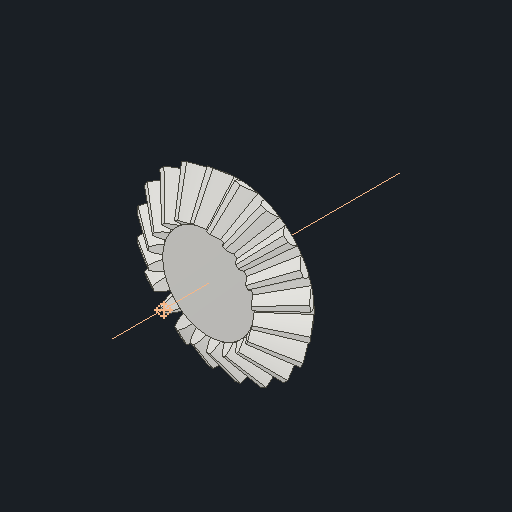
# Autodesk Inventor part: 베벨 기어1
Saved by Autodesk Inventor 2026.1 (Build 301233020, 233B)
## iProperties
Created: 2025-11-23
Part Number: 베벨 기어1
Material: Steel, Mild
Document SubType Name: Modeling
Designer: jaewook
Categories: <?xml version="1.0" encoding="UTF-16"?> <MemberInstance><Categories><FamilyTemplate><FamilyTemplateParameter ValueType="xs:double" Id="1" ObjectReferenceKey="da_z" ObjectType="kUserParameterObject"/><FamilyTemplateParameter ValueType="xs:double" Id="2" ObjectReferenceKey="da_b" ObjectType="kUserParameterObject"/><FamilyTemplateParameter ValueType="xs:double" Id="3" ObjectReferenceKey="da_beta" ObjectType="kUserParameterObject"/><FamilyTemplateParameter ValueType="xs:double" Id="4" ObjectReferenceKey="da_dae" ObjectType="kUserParameterObject"/><FamilyTemplateParameter ValueType="xs:double" Id="5" ObjectReferenceKey="da_ve" ObjectType="kUserParameterObject"/><FamilyTemplateParameter ValueType="xs:double" Id="6" ObjectReferenceKey="da_omega" ObjectType="kUserParameterObject"/><FamilyTemplateParameter ValueType="xs:string" Id="7" ObjectReferenceKey="EAIAABAAAAAAHwAAAAAAAIAAAAAAAAAA" ObjectType="83914240" SubObjectId="SurfaceGeometry"/></FamilyTemplate><ParamToTemplateMap><ParamToTemplate CategoryParameter="//CategoryParameter[@InternalName='046C89C9-8512-4d59-83FE-43B91F4F132A']" TemplateParameter="1"/><ParamToTemplate CategoryParameter="//CategoryParameter[@InternalName='2552DF32-E462-4b46-AEBF-C6C7768E72AC']" TemplateParameter="2"/><ParamToTemplate CategoryParameter="//CategoryParameter[@InternalName='C9EE641D-15FC-4fae-A226-E94C4372FDD7']" TemplateParameter="3"/><ParamToTemplate><ParamToTemplate CategoryParameter="//CategoryParameter[@InternalName='00B6519A-459B-49c7-AD84-2E56D39A5744']" ConstantValue="0.000000"/></ParamToTemplate><ParamToTemplate><ParamToTemplate CategoryParameter="//CategoryParameter[@InternalName='04B31F0E-C7A6-4894-AA32-9629BEFACF47']" ConstantValue="1.000000"/></ParamToTemplate><ParamToTemplate><ParamToTemplate CategoryParameter="//CategoryParameter[@InternalName='43CBEC2E-7847-49e7-A936-2F7889FCB2D9']" ConstantValue="0.200000"/></ParamToTemplate><ParamToTemplate><ParamToTemplate CategoryParameter="//CategoryParameter[@InternalName='B1EFC894-105D-4ebd-86BF-FA20ED196853']" ConstantValue="0.300000"/></ParamToTemplate><ParamToTemplate><ParamToTemplate CategoryParameter="//CategoryParameter[@InternalName='51175063-3D10-4879-93E8-6246FE8B403D']" ConstantValue="2060000000.000000"/></ParamToTemplate><ParamToTemplate><ParamToTemplate CategoryParameter="//CategoryParameter[@InternalName='A3A52E27-4454-46a9-B0BD-C932399B70AF']" ConstantValue="0.300000"/></ParamToTemplate><ParamToTemplate CategoryParameter="//CategoryParameter[@InternalName='2A200944-5A8C-41ca-B96E-8520D2E510F1']" TemplateParameter="4"/><ParamToTemplate><ParamToTemplate CategoryParameter="//CategoryParameter[@InternalName='1A637F62-92C8-44bc-B81F-10802510B579']" ConstantValue="1.594223"/></ParamToTemplate><ParamToTemplate CategoryParameter="//CategoryParameter[@InternalName='B52DD4BE-6863-48fb-BF58-89EF6F9EC65C']" TemplateParameter="5"/><ParamToTemplate><ParamToTemplate CategoryParameter="//CategoryParameter[@InternalName='3956BFF2-84D2-457d-93C2-9B0613DEBA67']" ConstantValue="0.541611"/></ParamToTemplate><ParamToTemplate CategoryParameter="//CategoryParameter[@InternalName='739CFA02-461B-4bf8-8049-181FCAD8B28F']" TemplateParameter="6"/><ParamToTemplate><ParamToTemplate CategoryParameter="//CategoryParameter[@InternalName='A27E999F-E2CE-4481-8A2A-EBF499C4C3C5']" ConstantValue="0.000000"/></ParamToTemplate><ParamToTemplate><ParamToTemplate CategoryParameter="//CategoryParameter[@InternalName='9E1B4470-B2D3-4ff1-B813-535BB4CDF51A']" ConstantValue="3520000.000000"/></ParamToTemplate><ParamToTemplate><ParamToTemplate CategoryParameter="//CategoryParameter[@InternalName='F8452263-BFF6-458c-9FB1-07C4B99E95CD']" ConstantValue="11400000.000000"/></ParamToTemplate><ParamToTemplate><ParamToTemplate CategoryParameter="//CategoryParameter[@InternalName='3E3BB259-FD49-497f-8171-6EBC954A3479']" ConstantValue="2.000000"/></ParamToTemplate><ParamToTemplate CategoryParameter="//CategoryParameter[@InternalName='27C3BAF2-7550-4e4b-AE2C-0DB134B7D9B7']" TemplateParameter="7"/></ParamToTemplateMap><Category DisplayName="Gear" InternalName="DC85795E-93AB-48d5-8EEE-5A27447B64BD" Mnemonic="Gear"><CategoryParameter DisplayName="z" InternalName="046C89C9-8512-4d59-83FE-43B91F4F132A" Mnemonic="z"/><CategoryParameter DisplayName="b" InternalName="2552DF32-E462-4b46-AEBF-C6C7768E72AC" Mnemonic="b"/><CategoryParameter DisplayName="||b|" InternalName="C9EE641D-15FC-4fae-A226-E94C4372FDD7" Mnemonic="beta"/><CategoryParameter DisplayName="x" InternalName="00B6519A-459B-49c7-AD84-2E56D39A5744" Mnemonic="x"/><CategoryParameter DisplayName="a*" InternalName="04B31F0E-C7A6-4894-AA32-9629BEFACF47" Mnemonic="a"/><CategoryParameter DisplayName="c*" InternalName="43CBEC2E-7847-49e7-A936-2F7889FCB2D9" Mnemonic="c"/><CategoryParameter DisplayName="r|.f|*" InternalName="B1EFC894-105D-4ebd-86BF-FA20ED196853" Mnemonic="rf"/><CategoryParameter DisplayName="E" InternalName="51175063-3D10-4879-93E8-6246FE8B403D" Mnemonic="E"/><CategoryParameter DisplayName="||m|" InternalName="A3A52E27-4454-46a9-B0BD-C932399B70AF" Mnemonic="mi"/><Category DisplayName="BevelGear" InternalName="0C98F69A-0C2B-4791-B2FE-7691BB227E77" Mnemonic="BevelGear"><CategoryParameter DisplayName="d|.ae|" InternalName="2A200944-5A8C-41ca-B96E-8520D2E510F1" Mnemonic="dae"/><CategoryParameter DisplayName="d|.ai|" InternalName="1A637F62-92C8-44bc-B81F-10802510B579" Mnemonic="dai"/><CategoryParameter DisplayName="A|.e|" InternalName="B52DD4BE-6863-48fb-BF58-89EF6F9EC65C" Mnemonic="ve"/><CategoryParameter DisplayName="A|.i|" InternalName="3956BFF2-84D2-457d-93C2-9B0613DEBA67" Mnemonic="vi"/><CategoryParameter DisplayName="||S|" InternalName="739CFA02-461B-4bf8-8049-181FCAD8B28F" Mnemonic="omega"/><CategoryParameter DisplayName="x|.t|" InternalName="A27E999F-E2CE-4481-8A2A-EBF499C4C3C5" Mnemonic="xt"/><CategoryParameter DisplayName="||s||.Flim|" InternalName="9E1B4470-B2D3-4ff1-B813-535BB4CDF51A" Mnemonic="sFlim"/><CategoryParameter DisplayName="||s||.Hlim|" InternalName="F8452263-BFF6-458c-9FB1-07C4B99E95CD" Mnemonic="sHlim"/><CategoryParameter DisplayName="유형" InternalName="3E3BB259-FD49-497f-8171-6EBC954A3479" Mnemonic="type"/><CategoryParameter DisplayName="PitchDiameter" InternalName="27C3BAF2-7550-4e4b-AE2C-0DB134B7D9B7" Mnemonic="IDS_PITCHDIAM"/></Category></Category></Categories></MemberInstance>
Mass: 60.9118 g
Surface Area: 34.3074 cm^2
Volume: 7.7496 cm^3
Density: 7.86 g/cm^3
Appearance: Steel
CustomPartVersion: 1
Author: jaewook
Autodesk Inventor part; units mm, degrees
ref_plane "메쉬 평면2" through (0, 0, 0) normal (0.9876883, 0.1564345, 0) x (0, 0, 1)
sketch "톱니 본체 스케치" plane through (0, 0, 0) normal (1, 0, 0) x (0, 1, 0)
  line L0 (0, 0) -> (11.562957, -11.171303) construction
  line L1 (11.562957, -11.171303) -> (13.280869, -9.023914)
  line L2 (13.280869, -9.023914) -> (0, 0) construction
  line L3 (12.5, -10) -> (0, 0) construction
  line L4 (6.940031, -6.704962) -> (7.971113, -5.41611)
  line L5 (11.562957, -11.171303) -> (6.940031, -6.704962)
  line L6 (13.280869, -9.023914) -> (7.971113, -5.41611)
  line L7 (0, -39.386751) -> (0, 6.564458)
  line L8 (0, -10) -> (13.280869, -10) construction
  dimension "d0" = 25
  dimension "d1" = 23.12591
  dimension "d2" = 26.56174
  dimension "d3" = 6.4
  dimension "d4" = 9.02391
  constraints: 16 end point, 4 point on line, 3 perpendicular, 2 collinear, 1 horizontal alignment, 1 vertical alignment
  measures "d0" diameter of L3.start L7
  measures "d1" diameter of L0.end L7
  measures "d2" diameter of L1.end L7
  measures "d3" distance between parallel lines of L1 L4
  measures "d4" vertical distance of L1.end L0.start
revolve "톱니 본체" add sketch "톱니 본체 스케치" angle 360 about axis through (0, 0, 0) along (0, 0, 1)
ref_plane "톱니 평면" through (0, 12.5, -10) normal (0, -0.7808688, 0.624695) x (1, 0, 0)
sketch "시작 스케치" plane through (0, 12.5, -10) normal (0, -0.7808688, 0.624695) x (1, 0, 0)
  line L0 (0, -23.505131) -> (0, 10.644758)
  arc A0 (-0.488954, -1.83) -> (-2.245942, 1.960501) centre (-7.685775, -2.863445) ccw
  arc A1 (2.245942, 1.960501) -> (0.488954, -1.83) centre (7.685775, -2.863445) ccw
  line L1 (-0.488954, -1.83) -> (0.488954, -1.83)
  arc A2 (2.245942, 1.960501) -> (-2.245942, 1.960501) centre (0, -20.009763) ccw
  dimension "d7" = 7.27064
  dimension "d8" = 7.68577
  dimension "d9" = 17.14632
  dimension "d57" = 22.08476
  dimension "d58" = 18.17976
  constraints: 6 point on circle, 3 centre point, 3 symmetric about line, 2 end point, 1 coincident, 1 perpendicular, 1 other
  measures "d7" radius of A0
  measures "d8" horizontal distance of point (0, -20.01) A0.centre
  measures "d9" vertical distance of point (0, -20.01) A0.centre
  measures "d57" radius of A2
  measures "d58" distance from line of A2.centre L1
ref_plane "끝 평면" through (0, 7.39507, -5.916056) normal (0, -0.7808688, 0.624695) x (1, 0, 0)
sketch "끝 스케치" plane through (0, 7.39507, -5.916056) normal (0, -0.7808688, 0.624695) x (1, 0, 0)
  line L0 (0, -15.35404) -> (0, 6.953444)
  arc A0 (-0.289268, -1.082638) -> (-1.328712, 1.159843) centre (-4.546948, -1.69403) ccw
  arc A1 (1.328712, 1.159843) -> (0.289268, -1.082638) centre (4.546948, -1.69403) ccw
  line L1 (-0.289268, -1.082638) -> (0.289268, -1.082638)
  arc A2 (1.328712, 1.159843) -> (-1.328712, 1.159843) centre (0, -11.837888) ccw
  dimension "d12" = 4.30135
  dimension "d15" = 4.54695
  dimension "d16" = 10.14386
  dimension "d59" = 13.06547
  dimension "d60" = 10.75525
  constraints: 6 point on circle, 3 centre point, 3 symmetric about line, 2 end point, 1 coincident, 1 other
  measures "d12" radius of A0
  measures "d15" horizontal distance of A0.centre point (0, -11.838)
  measures "d16" vertical distance of A0.centre point (0, -11.838)
  measures "d59" radius of A2
  measures "d60" distance from line of A2.centre L1
loft "Loft" cut profiles "시작 스케치", "끝 스케치"
pattern_circular "Circular Pattern" count 20 over 360 about axis through (0, 0, 0) along (0, 0, 1) of "Loft"
sketch3d "3D 스케치 오른쪽"
ref_plane "끝 평면 오른쪽" through (-1.742858, 7.186759, -5.916056) normal (0.1840339, -0.7588726, 0.624695) x (0.9718311, 0.2356783, 0)
sketch "끝 스케치 오른쪽" plane through (-1.742858, 7.186759, -5.916056) normal (0.1840339, -0.7588726, 0.624695) x (0.9718311, 0.2356783, 0)
  arc A0 (-0.289268, -1.082638) -> (-1.328712, 1.159843) centre (-4.546948, -1.69403) ccw
  line L0 (0, -17.993564) -> (0, 9.592957)
  arc A1 (1.328712, 1.159843) -> (0.289268, -1.082638) centre (4.546948, -1.69403) ccw
  line L1 (-0.289268, -1.082638) -> (0.289268, -1.082638)
  arc A2 (1.328712, 1.159843) -> (-1.328712, 1.159843) centre (0, -11.837888) ccw
  dimension "d70" = 4.54695
  dimension "d71" = 10.14386
  dimension "d72" = 4.30135
  dimension "d73" = 10.75525
  dimension "d74" = 13.06547
  constraints: 6 point on circle, 3 centre point, 3 symmetric about line, 2 end point, 1 coincident, 1 perpendicular, 1 other
  measures "d70" horizontal distance of A2.centre A0.centre
  measures "d71" vertical distance of point (0, -11.838) A0.centre
  measures "d72" radius of A0
  measures "d73" distance from line of point (0, -11.838) L1
  measures "d74" radius of A2
feature "로프트 오른쪽" [suppressed]
pattern_circular "원형 패턴 오른쪽" [suppressed]
sketch3d "3D 스케치 왼쪽"
ref_plane "끝 평면 왼쪽" through (1.76116, 7.186759, -5.923915) normal (-0.1858037, -0.7582085, 0.6249775) x (0.9712618, -0.2380138, 0)
sketch "끝 스케치 왼쪽" plane through (1.76116, 7.186759, -5.923915) normal (-0.1858037, -0.7582085, 0.6249775) x (0.9712618, -0.2380138, 0)
  line L0 (0, -31.02314) -> (0, 14.000417)
  arc A0 (-0.289268, -1.079211) -> (-1.328712, 1.16327) centre (-4.546948, -1.690603) ccw
  arc A1 (1.328712, 1.16327) -> (0.289268, -1.079211) centre (4.546948, -1.690603) ccw
  line L1 (-0.289268, -1.079211) -> (0.289268, -1.079211)
  ellipse E0 centre (0, -4.228047) end of major axis (7.971113, -4.228047) minor radius 4.981766
  arc A2 (1.328712, 1.16327) -> (-1.328712, 1.16327) centre (0, -11.834461) ccw
  dimension "d56" = 4.98177
  dimension "d30" = 4.30135
  dimension "d31" = 4.54695
  dimension "d32" = 10.14386
  dimension "d61" = 13.06547
  dimension "d62" = 10.75525
  constraints: 6 point on circle, 3 centre point, 3 symmetric about line, 2 end point, 1 coincident, 2 other
  measures "d30" radius of A0
  measures "d31" horizontal distance of point (0, -11.834) A0.centre
  measures "d32" vertical distance of A0.centre point (0, -11.834)
  measures "d61" radius of A2
  measures "d62" distance from line of point (0, -11.834) L1
feature "로프트 왼쪽" [suppressed]
pattern_circular "원형 패턴 왼쪽" [suppressed]
sketch "본체 스케치" plane through (0, 0, 0) normal (1, 0, 0) x (0, 1, 0)
  line L0 (0, -35.037536) -> (0, -19.530831)
  line L1 (11.562957, -11.171303) -> (6.940031, -6.704962)
  line L2 (6.940031, -6.704962) -> (0, -6.704962)
  line L3 (11.562957, -11.171303) -> (0, -11.171303)
  constraints: 4 end point, 2 perpendicular, 2 point on line
sketch "본체 스케치 outline for 본체 고정" plane through (0, 0, 0) normal (1, 0, 0) x (0, 1, 0)
  line L0 (0, -11.171303) -> (11.562957, -11.171303)
  line L1 (0, -6.704962) -> (0, -11.171303)
  line L2 (6.940031, -6.704962) -> (0, -6.704962)
  line L3 (11.562957, -11.171303) -> (6.940031, -6.704962)
revolve "본체 고정" add sketch "본체 스케치 outline for 본체 고정" angle 360 about axis through (0, 0, 0) along (0, 0, 1)
sketch "Sketch6" plane through (0, 0, 0) normal (1, 0, 0) x (0, 1, 0)
  line L0 (12.5, -10) -> (0, 0)
  line L1 (0, -37.799919) -> (0, 6.299986)
surface revolve "피치 지름" sketch "Sketch6" angle 360 about axis through (0, 0, 0) along (0, 0, 1) shown no curves L0
equation "\"d0\" = da_de"
equation "\"d1\" = da_dfe"
equation "\"d2\" = da_dae"
equation "\"d3\" = da_b"
equation "\"d4\" = da_ve"
equation "\"d7\" = fd_rr"
equation "\"d8\" = fd_x"
equation "\"d9\" = fd_y"
equation "\"d57\" = 0.5 * fd_dva + 0.3 * da_he"
equation "\"d58\" = 0.5 * fd_dva - 1.12 * da_he"
equation "\"da_teethtype\" = 0"
equation "\"da_b\" = 6.4"
equation "\"da_de\" = 25"
equation "\"da_dae\" = 26.56174"
equation "\"da_dfe\" = 23.12591"
equation "\"da_le\" = 16.00781"
equation "\"da_omega\" = 90deg"
equation "\"da_beta\" = 0"
equation "\"da_delta\" = 51.340192deg"
equation "\"da_alpha\" = 20deg"
equation "\"da_he\" = 2.75"
equation "\"da_ve\" = 9.02391"
equation "\"da_zv\" = 32.015621"
equation "\"fd_loft\" = da_b + 0.05 * da_he"
equation "\"fd_x\" = fd_x1 + fd_x2"
equation "\"fd_y\" = fd_y1 - fd_y2"
equation "\"fd_dd\" = fd_dva - 0.8 * da_he"
equation "\"da_dvw\" = 40.01953"
equation "\"d11\" = fd_loft"
equation "\"da_dm\" = 20.00244"
equation "\"da_x\" = 0"
equation "\"da_m\" = 1.25"
equation "\"d50\" = da_omega"
equation "\"fd_rr\" = 7.270642"
equation "\"fd_dva\" = 42.519526"
equation "\"fd_x1\" = 0.992249"
equation "\"fd_x2\" = 6.693526"
equation "\"fd_y1\" = 19.985146"
equation "\"fd_y2\" = 2.838828"
body "Solid1"
body "Srf1"
